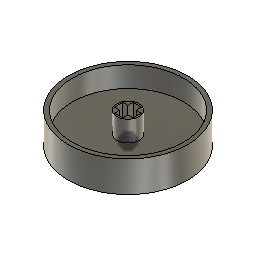
ControllerCaps (Autodesk Fusion 360 design; units mm, degrees)
Autodesk Fusion 360 part; units mm, degrees
sketch "Sketch1" plane through (0, 0, 0) normal (0, 0, 1) x (1, 0, 0)
sketch "Sketch2" plane through (0, 0, 0) normal (0, 0, 1) x (1, 0, 0)
cylinder "CylinderPrimitive4" add diameter 5.4 height 6.5 placed x (1, 0, 0) y (0, 1, 0) z (0, 0, 1) at (0, 0, 0) makes body 1
box "BoxPrimitive3" add length 0.5 width 2 height 1 placed x (0, -1, 0) y (1, 0, 0) z (0, 0, 1) at (0, 0, 6.5) separate body makes body 2
box "BoxPrimitive4" add length 0.5 width 2 height 1 placed x (0, 1, 0) y (-1, 0, 0) z (0, 0, 1) at (2, 0, 6.5) separate body makes body 3
box "BoxPrimitive5" add length 0.5 width 2 height 1 placed x (0, -1, 0) y (1, 0, 0) z (0, 0, 1) at (-2, 0, 6.5) separate body makes body 4
box "BoxPrimitive6" add length 0.5 width 2 height 1 placed x (0, 1, 0) y (-1, 0, 0) z (0, 0, 1) at (0, 0, 6.5) separate body makes body 5
box "BoxPrimitive7" add length 2 width 0.5 height 1 placed x (0, 1, 0) y (-1, 0, 0) z (0, 0, 1) at (0.5, 0, 6.5) separate body makes body 6
box "BoxPrimitive8" add length 2 width 0.5 height 1 placed x (0, 1, 0) y (-1, 0, 0) z (0, 0, 1) at (0, 0, 6.5) separate body makes body 7
box "BoxPrimitive9" add length 2 width 0.5 height 1 placed x (0, -1, 0) y (1, 0, 0) z (0, 0, 1) at (0, 0, 6.5) separate body makes body 8
box "BoxPrimitive10" add length 2 width 0.5 height 1 placed x (0, -1, 0) y (1, 0, 0) z (0, 0, 1) at (-0.5, 0, 6.5) separate body makes body 9
combine "Combine1" operation add target body 2 tool bodies 3 4 5 6 7 8 9
cylinder "CylinderPrimitive5" add diameter 29 height 1.5 placed x (1, 0, 0) y (0, 1, 0) z (0, 0, 1) at (0, 0, 0) separate body makes body 10
extrude "Extrude2" add 1 faces at (-4.1542, 3.427, 0) along direction (0, 0, -1) blind 1 on bodies 10 bodies 1 2 10
extrude "Extrude3" cut 1 faces at (-1, 0.1667, 7.5) along direction (0, 0, -1) blind 7.5 on bodies 2 bodies 1 2
cylinder "CylinderPrimitive6" add diameter 29 height 5 placed x (1, 0, 0) y (0, 1, 0) z (0, 0, 1) at (0, 0, 0) separate body makes body 11
move_body "Move3" bodies 11 to x (1, 0, 0) y (0, 1, 0) z (0, 0, 1) at (0, 0, 1)
move_body "Move4" bodies 11 to x (1, 0, 0) y (0, 1, 0) z (0, 0, 1) at (0, 0, 0.5)
shell "Shell1" thickness 1 removed faces 1 at (-4.1542, 3.427, 6.5) on bodies 11
extrude "Extrude4" cut 1 faces at (-0.606, -3.1054, 2.5) along direction (0, 0, -1) blind 1 on bodies 11 bodies 11
combine "Combine2" operation add target body 11 tool bodies 1
extrude "Extrude5" add 1 faces at (-1, 0.1667, 0) along direction (0, 0, 1) blind 6.5 on bodies 11 bodies 2 11
box "BoxPrimitive11" add length 2 width 1 height 0.5 placed x (0, 1, 0) y (-1, 0, 0) z (0, 0, 1) at (0, 0, 6.5) bodies 2
box "BoxPrimitive12" add length 2 width 1 height 0.5 placed x (0, 1, 0) y (-1, 0, 0) z (0, 0, 1) at (1, 0, 6.5) bodies 2
box "BoxPrimitive13" add length 2 width 1 height 0.5 placed x (0, -1, 0) y (1, 0, 0) z (0, 0, 1) at (-1, 0, 6.5) bodies 2
box "BoxPrimitive14" add length 2 width 1 height 0.5 placed x (0, -1, 0) y (1, 0, 0) z (0, 0, 1) at (0, 0, 6.5) bodies 2
box "BoxPrimitive15" add length 1 width 2 height 0.5 placed x (0, 1, 0) y (-1, 0, 0) z (0, 0, 1) at (0, 0, 6.5) bodies 2
box "BoxPrimitive16" add length 1 width 2 height 0.5 placed x (0, -1, 0) y (1, 0, 0) z (0, 0, 1) at (-2, 0, 6.5) bodies 2
box "BoxPrimitive17" add length 1 width 2 height 0.5 placed x (0, 1, 0) y (-1, 0, 0) z (0, 0, 1) at (2, 0, 6.5) bodies 2
box "BoxPrimitive18" add length 1 width 2 height 0.5 placed x (0, -1, 0) y (1, 0, 0) z (0, 0, 1) at (0, 0, 6.5) bodies 2
extrude "Extrude6" cut 1 faces at (-0.3333, -0.3333, 7) along direction (0, 0, -1) blind 7 on bodies 2 bodies 2
extrude "Extrude7" cut 1 faces at (-2, 0.3333, 4.3333) along direction (-1, 0, 0) blind 0.25 on bodies 2 bodies 2
extrude "Extrude8" cut 1 faces at (0.3333, -2, 4.3333) along direction (0, -1, 0) blind 0.25 on bodies 2 bodies 2
extrude "Extrude9" cut 1 faces at (2, -0.3333, 4.3333) along direction (1, 0, 0) blind 0.25 on bodies 2 bodies 2
extrude "Extrude10" cut 1 faces at (0.3333, 2, 4.3333) along direction (0, 1, 0) blind 0.25 on bodies 2 bodies 2
